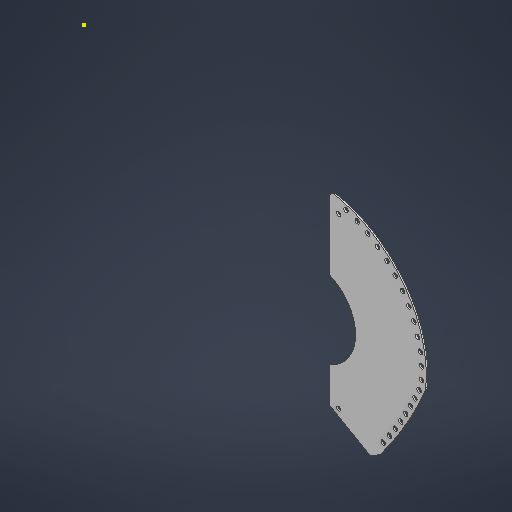
# Autodesk Inventor part: TopCurve
Saved by Autodesk Inventor 2026.1 (Build 301233000, 233)
## iProperties
Created: 2026-03-09
Part Number: TopCurve
Material: Generic
Document SubType Name: Modeling
Designer: roejo
Density: 1 g/cm^3
Appearance: Default
Author: roejo
Autodesk Inventor part; units mm, degrees
ref_plane "YZ Plane" through (0, 0, 0) normal (1, 0, 0) x (0, 1, 0)
ref_plane "XZ Plane" through (0, 0, 0) normal (0, 1, 0) x (-1, 0, 0)
ref_plane "XY Plane" through (0, 0, 0) normal (0, 0, 1) x (1, 0, 0)
sketch "Sketch1" plane through (0, 0, 0) normal (0, 0, 1) x (1, 0, 0)
  circle A0 centre (241.6154, -140.1465) radius 2.4638
  arc A1 (259.0779, -181.0227) -> (259.0779, -99.2703) centre (241.6154, -140.1465) ccw
  line L0 (259.0779, -218.2466) -> (259.0779, -181.0227)
  arc A2 (312.3724, -235.9031) -> (359.2204, -154.9095) centre (11.2573, -7.6879) ccw
  arc A3 (359.2204, -154.9095) -> (360.17, -151.1328) centre (347.5241, -149.9609) ccw
  arc A4 (360.17, -151.1328) -> (262.8183, -22.9871) centre (241.6154, -140.1465) ccw
  arc A5 (301.8563, -242.8447) -> (312.3724, -235.9031) centre (241.6154, -140.1465) ccw
  arc A6 (262.8183, -22.9871) -> (259.0779, -26.1114) centre (262.2529, -26.1114) ccw
  line L1 (259.0779, -26.1114) -> (259.0779, -99.2703)
  line L2 (259.0779, -181.0227) -> (259.0779, -218.2466)
  circle A7 centre (268.2854, -38.5465) radius 2.1844
  circle A8 centre (268.2854, -216.3465) radius 2.1844
  arc A9 (308.9934, -232.4758) -> (354.8343, -153.0538) centre (11.2573, -7.6879) ccw
  arc A10 (354.8343, -153.0538) -> (355.4278, -150.6933) centre (347.5241, -149.9609) ccw
  arc A11 (355.4278, -150.6933) -> (263.8404, -28.0281) centre (241.6154, -140.1465) ccw
  circle A12 centre (263.8404, -28.0281) radius 2.413
  circle A13 centre (276.0241, -31.1486) radius 2.413
  circle A14 centre (287.7911, -35.5889) radius 2.413
  circle A15 centre (298.9991, -41.2951) radius 2.413
  circle A16 centre (309.5123, -48.1981) radius 2.413
  circle A17 centre (319.2034, -56.2144) radius 2.413
  circle A18 centre (327.9551, -65.247) radius 2.413
  circle A19 centre (335.6615, -75.1863) radius 2.413
  circle A20 centre (342.2292, -85.9122) radius 2.413
  circle A21 centre (347.5787, -97.2948) radius 2.413
  circle A22 centre (351.6452, -109.1961) radius 2.413
  circle A23 centre (354.3796, -121.4722) radius 2.413
  circle A24 centre (355.7487, -133.9744) radius 2.413
  circle A25 centre (355.7358, -146.5513) radius 2.413
  circle A26 centre (353.0365, -157.2317) radius 2.413
  circle A27 centre (348.7088, -166.7567) radius 2.413
  circle A28 centre (344.0523, -176.2817) radius 2.413
  circle A29 centre (339.0531, -185.8067) radius 2.413
  circle A30 centre (333.6952, -195.3317) radius 2.413
  circle A31 centre (327.9604, -204.8567) radius 2.413
  circle A32 centre (321.8278, -214.3817) radius 2.413
  circle A33 centre (315.2734, -223.9067) radius 2.413
  line L3 (301.8563, -242.8447) -> (259.0779, -218.2466)
  point P0 (259.0779, -22.3716)
  point P1 (295.3179, -246.41)
  dimension "d4" = 88.9
  dimension "d5" = 12.7
  dimension "d7" = 4.3688
  dimension "d8" = 4.7625
  dimension "d9" = 4.826
  dimension "d12" = 82
  dimension "d14" = 4.826
  dimension "d21" = 4.826
  dimension "d22" = 4.826
  dimension "d23" = 4.826
  dimension "d24" = 4.826
  dimension "d25" = 4.826
  dimension "d26" = 4.826
  dimension "d27" = 4.826
  dimension "d28" = 9.525
  dimension "d29" = 9.525
  dimension "d30" = 9.525
  dimension "d31" = 9.525
  dimension "d32" = 9.525
  dimension "d33" = 9.525
  dimension "d34" = 9.525
  dimension "d41" = 177.8
  dimension "d42" = 9.2075
  constraints: 33 centre point, 18 point on circle, 8 end point, 4 tangent, 3 coincident, 45 other
  measures "d4" diameter of A1
  measures "d5" radius of A3
  measures "d7" diameter of A8
  measures "d8" radial gap between concentric circles of A4 A11
  measures "d9" diameter of A12
  measures "d14" diameter of A26
  measures "d21" diameter of A27
  measures "d22" diameter of A28
  measures "d23" diameter of A29
  measures "d24" diameter of A30
  measures "d25" diameter of A31
  measures "d26" diameter of A32
  measures "d27" diameter of A33
  measures "d28" vertical distance of A27.centre A26.centre
  measures "d29" vertical distance of A28.centre A27.centre
  measures "d30" vertical distance of A29.centre A28.centre
  measures "d31" vertical distance of A30.centre A29.centre
  measures "d32" vertical distance of A31.centre A30.centre
  measures "d33" vertical distance of A32.centre A31.centre
  measures "d34" vertical distance of A32.centre A33.centre
  measures "d41" distance of A8.centre A7.centre
  measures "d42" distance from line of L1 A7.centre
extrude "Extrusion1" add sketch "Sketch1" along normal blind 1.5875 contours A1 L1 A6 A4 A3 A2 A5 L3 L0
sketch "Sketch4" plane through (0, 0, 1.5875) normal (0, 0, 1) x (1, 0, 0)
  point P0 (0, 0)
sketch "Sketch5" plane through (0, 0, 1.5875) normal (0, 0, 1) x (1, 0, 0)
  arc A0 (359.2204, -154.9095) -> (360.17, -151.1328) centre (347.5241, -149.9609) ccw projected
  arc A1 (360.17, -151.1328) -> (262.8183, -22.9871) centre (241.6154, -140.1465) ccw projected
  arc A2 (262.8183, -22.9871) -> (259.0779, -26.1114) centre (262.2529, -26.1114) ccw projected
  line L0 (259.0779, -26.1114) -> (259.0779, -99.2703) projected
  arc A3 (259.0779, -181.0227) -> (259.0779, -99.2703) centre (241.6154, -140.1465) ccw projected
  line L1 (259.0779, -181.0227) -> (259.0779, -218.2466) projected
  line L2 (259.0779, -218.2466) -> (301.8563, -242.8447) projected
  arc A4 (301.8563, -242.8447) -> (312.3724, -235.9031) centre (241.6154, -140.1465) ccw projected
  arc A5 (312.3724, -235.9031) -> (359.2204, -154.9095) centre (11.2573, -7.6879) ccw projected
  circle A6 centre (263.8404, -28.0281) radius 2.413 projected
  circle A7 centre (276.0241, -31.1486) radius 2.413 projected
  circle A8 centre (287.7911, -35.5889) radius 2.413 projected
  circle A9 centre (298.9991, -41.2951) radius 2.413 projected
  circle A10 centre (309.5123, -48.1981) radius 2.413 projected
  circle A11 centre (319.2034, -56.2144) radius 2.413 projected
  circle A12 centre (327.9551, -65.247) radius 2.413 projected
  circle A13 centre (335.6615, -75.1863) radius 2.413 projected
  circle A14 centre (342.2292, -85.9122) radius 2.413 projected
  circle A15 centre (347.5787, -97.2948) radius 2.413 projected
  circle A16 centre (351.6452, -109.1961) radius 2.413 projected
  circle A17 centre (354.3796, -121.4722) radius 2.413 projected
  circle A18 centre (355.7487, -133.9744) radius 2.413 projected
  circle A19 centre (355.7358, -146.5513) radius 2.413 projected
  circle A20 centre (353.0365, -157.2317) radius 2.413 projected
  circle A21 centre (348.7088, -166.7567) radius 2.413 projected
  circle A22 centre (344.0523, -176.2817) radius 2.413 projected
  circle A23 centre (339.0531, -185.8067) radius 2.413 projected
  circle A24 centre (333.6952, -195.3317) radius 2.413 projected
  circle A25 centre (327.9604, -204.8567) radius 2.413 projected
  circle A26 centre (321.8278, -214.3817) radius 2.413 projected
  circle A27 centre (268.2854, -38.5465) radius 2.1844 projected
  circle A28 centre (315.2734, -223.9067) radius 2.413 projected
  circle A29 centre (268.2854, -216.3465) radius 2.1844 projected
  circle A30 centre (263.8404, -28.0281) radius 2.413
  point P0 (0, 0)
  constraints: 1 centre point, 1 coincident, 1 concentric
extrude "Extrusion3" add sketch "Sketch5" against normal blind 1.5875 contours A6
body "Solid1"
